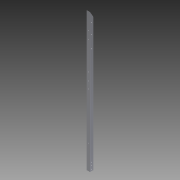
# Autodesk Inventor part: 1x1 support
Saved by Autodesk Inventor 2015 (Build 190159000, 159)
## iProperties
Created: 2015-01-17
Part Number: 1x1 support
Material: Aluminum 6061
Document SubType Name: Modeling
Designer: Jarod
Density: 2.7 g/cm^3
Appearance: Aluminum - Flat
Author: Jarod
Autodesk Inventor part; units mm, degrees
ref_plane "YZ Plane" through (0, 0, 0) normal (1, 0, 0) x (0, 1, 0)
ref_plane "XZ Plane" through (0, 0, 0) normal (0, 1, 0) x (-1, 0, 0)
ref_plane "XY Plane" through (0, 0, 0) normal (0, 0, 1) x (1, 0, 0)
sketch "Sketch1" plane through (0, 0, 0) normal (0, 1, 0) x (-1, 0, 0)
  line L0 (0, 0) -> (25.4, 0)
  line L1 (25.4, 0) -> (25.4, -25.4)
  line L2 (25.4, -25.4) -> (0, -25.4)
  line L3 (0, -25.4) -> (0, 0)
  line L4 (3.175, -3.175) -> (22.225, -3.175)
  line L5 (22.225, -3.175) -> (22.225, -22.225)
  line L6 (22.225, -22.225) -> (3.175, -22.225)
  line L7 (3.175, -22.225) -> (3.175, -3.175)
  dimension "d0" = 25.4
  dimension "d1" = 25.4
  dimension "d2" = 19.05
  dimension "d3" = 19.05
  dimension "d4" = 3.175
  dimension "d5" = 3.175
  constraints: 16 end point, 4 parallel, 2 horizontal, 2 perpendicular
  measures "d0" distance of L1.end L2.end
  measures "d1" distance of L0.end L1.end
  measures "d2" distance of L5.end L6.end
  measures "d3" distance of L4.end L5.end
  measures "d4" distance between parallel lines of L3 L7
  measures "d5" distance between parallel lines of L0 L4
extrude "Extrusion1" add sketch "Sketch1" along normal blind 1012.825
sketch "Sketch2" plane through (-25.4, 0, -25.4) normal (-1, 0, 0) x (0, 0, 1)
  line L0 (25.4, 0) -> (0, 0) projected
  line L1 (25.4, 0) -> (25.4, 1012.825) projected
  line L2 (0, 1012.825) -> (25.4, 1012.825) projected
  line L3 (0, 0) -> (0, 1012.825) projected
  point P0 (12.7, 12.7)
  point P1 (12.7, 38.1)
  dimension "d8" = 12.7
  dimension "d9" = 38.1
  dimension "d14" = 12.7
  dimension "d15" = 12.7
  measures "d8" distance from line of L0 point (12.7, 12.7)
  measures "d9" distance from line of point (12.7, 38.1) L0
  measures "d14" distance from line of L3 point (12.7, 12.7)
  measures "d15" distance from line of L3 point (12.7, 38.1)
hole "Hole1" at (-25.4, 12.7, -12.7) at (-25.4, 38.1, -12.7) direction (1, 0, 0) diameter 6.35 end through all
sketch "Sketch3" plane through (-25.4, 0, -25.4) normal (-1, 0, 0) x (0, 0, 1)
  circle A0 centre (12.7, 12.7) radius 3.175 projected
  circle A1 centre (12.7, 38.1) radius 3.175 projected
  line L0 (25.4, 0) -> (0, 0) projected
  line L1 (25.4, 0) -> (25.4, 1012.825) projected
  line L2 (0, 1012.825) -> (25.4, 1012.825) projected
  line L3 (0, 0) -> (0, 1012.825) projected
  line L4 (25.4, 1012.825) -> (0, 1012.825)
  line L5 (0, 1012.825) -> (0, 968.8309)
  line L6 (0, 0) -> (0, 1012.825) projected
  line L7 (0, 968.8309) -> (25.4, 1012.825)
  dimension "d57" = 60
  constraints: 6 end point, 1 horizontal, 1 point on line
  measures "d57" angle of L7 L2
extrude "Extrusion2" cut sketch "Sketch3" against normal blind 25.4 contours L7 L3 L2
sketch "Sketch5" plane through (-25.4, 0, -25.4) normal (-1, 0, 0) x (0, 0, 1)
  line L0 (25.4, 0) -> (0, 0) projected
  line L1 (25.4, 0) -> (25.4, 1012.825) projected
  point P0 (12.7, 774.7)
  dimension "d58" = 12.7
  dimension "d59" = 774.7
  measures "d58" distance from line of L1 point (12.7, 774.7)
  measures "d59" distance from line of L0 point (12.7, 774.7)
hole "Hole5" at (-25.4, 774.7, -12.7) direction (1, 0, 0) diameter 6.35 end through all
sketch "Sketch6" plane through (-25.4, 0, -25.4) normal (-1, 0, 0) x (0, 0, 1)
  line L0 (0, 0) -> (0, 968.8309) projected
  line L1 (25.4, 0) -> (0, 0) projected
  point P0 (12.7, 939.8)
  point P1 (12.7, 863.6)
  dimension "d67" = 12.7
  dimension "d68" = 12.7
  dimension "d69" = 863.6
  dimension "d70" = 939.8
  measures "d67" distance from line of L0 point (12.7, 939.8)
  measures "d68" distance from line of L0 point (12.7, 863.6)
  measures "d69" distance from line of L1 point (12.7, 863.6)
  measures "d70" distance from line of L1 point (12.7, 939.8)
hole "Hole6" at (-25.4, 939.8, -12.7) at (-25.4, 863.6, -12.7) direction (1, 0, 0) diameter 6.35 end through all
sketch "Sketch10" plane through (-25.4, 0, 0) normal (0, 0, 1) x (1, 0, 0)
  line L0 (25.4, 0) -> (0, 0) projected
  line L1 (0, 0) -> (0, 1012.825) projected
  point P0 (12.7, 628.65)
  point P1 (12.7, 571.5)
  point P2 (12.7, 520.7)
  point P3 (12.7, 889)
  point P4 (12.7, 831.85)
  point P5 (12.7, 177.8)
  dimension "d114" = 12.7
  dimension "d115" = 12.7
  dimension "d116" = 889
  dimension "d117" = 831.85
  dimension "d118" = 571.5
  dimension "d119" = 628.65
  dimension "d120" = 12.7
  dimension "d121" = 12.7
  dimension "d122" = 12.7
  dimension "d123" = 520.7
  dimension "d124" = 177.8
  dimension "d125" = 12.7
  measures "d114" distance from line of L1 point (12.7, 889)
  measures "d115" distance from line of L1 point (12.7, 831.85)
  measures "d116" distance from line of L0 point (12.7, 889)
  measures "d117" distance from line of L0 point (12.7, 831.85)
  measures "d118" distance from line of L0 point (12.7, 571.5)
  measures "d119" distance from line of L0 point (12.7, 628.65)
  measures "d120" distance from line of L1 point (12.7, 628.65)
  measures "d121" distance from line of L1 point (12.7, 571.5)
  measures "d122" distance from line of L1 point (12.7, 520.7)
  measures "d123" distance from line of L0 point (12.7, 520.7)
  measures "d124" distance from line of L0 point (12.7, 177.8)
  measures "d125" distance from line of L1 point (12.7, 177.8)
hole "Hole10" at (-12.7, 628.65, 0) at (-12.7, 571.5, 0) at (-12.7, 520.7, 0) at (-12.7, 889, 0) at (-12.7, 831.85, 0) at (-12.7, 177.8, 0) direction (0, 0, -1) diameter 6.35 end through all
sketch "Sketch11" plane through (-25.4, 0, -25.4) normal (-1, 0, 0) x (0, 0, 1)
  circle A0 centre (12.7, 939.8) radius 3.175 projected
  circle A1 centre (12.7, 863.6) radius 3.175 projected
  circle A2 centre (12.7, 774.7) radius 3.175 projected
  line L0 (25.4, 1012.825) -> (0, 968.8309) projected
  line L1 (0, 0) -> (0, 968.8309) projected
  line L2 (25.4, 0) -> (0, 0) projected
  line L3 (25.4, 0) -> (25.4, 1012.825) projected
  circle A3 centre (12.7, 38.1) radius 3.175 projected
  circle A4 centre (12.7, 12.7) radius 3.175 projected
  point P0 (12.7, 57.15)
  dimension "d133" = 57.15
  dimension "d134" = 12.7
  measures "d133" distance from line of L2 point (12.7, 57.15)
  measures "d134" distance from line of L1 point (12.7, 57.15)
hole "Hole11" at (-25.4, 57.15, -12.7) direction (1, 0, 0) diameter 6.35 end through all
body "Solid1"
